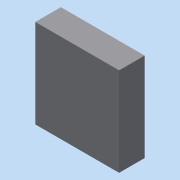
# Autodesk Inventor part: battery case
Saved by Autodesk Inventor 2015 (Build 190159000, 159)
## iProperties
Created: 2015-06-23
Part Number: battery case
Material: Generic
Document SubType Name: Modeling
Designer: Rahul
Density: 1 g/cm^3
Appearance: Default
Author: Rahul
Autodesk Inventor part; units mm, degrees
ref_plane "YZ Plane" through (0, 0, 0) normal (1, 0, 0) x (0, 1, 0)
ref_plane "XZ Plane" through (0, 0, 0) normal (0, 1, 0) x (-1, 0, 0)
ref_plane "XY Plane" through (0, 0, 0) normal (0, 0, 1) x (1, 0, 0)
sketch "Sketch1" plane through (0, 0, 0) normal (0, 0, 1) x (1, 0, 0)
  line L0 (-48.4452, 27.5932) -> (16.0708, 27.5932)
  line L1 (16.0708, 27.5932) -> (16.0708, -40.7328)
  line L2 (16.0708, -40.7328) -> (-48.4452, -40.7328)
  line L3 (-48.4452, -40.7328) -> (-48.4452, 27.5932)
  line L4 (-19.8209, 25.7702) -> (-12.7814, 25.7702) construction
  line L5 (-12.7814, 25.7702) -> (-12.7814, 20.739) construction
  line L6 (-12.7814, 20.739) -> (-19.8209, 20.739) construction
  line L7 (-19.8209, 20.739) -> (-19.8209, 25.7702) construction
  point P0 (0, 0)
  dimension "d0" = 68.326
  dimension "d1" = 64.516
  constraints: 8 end point, 2 parallel, 1 horizontal, 1 perpendicular, 2 other
  measures "d0" distance of L0.end L1.end
  measures "d1" distance of L0.start L0.end
extrude "Extrusion1" add sketch "Sketch1" against normal blind 19.685
body "Solid1"
